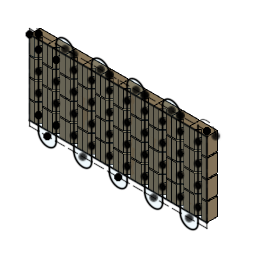
model (Autodesk Fusion 360 design; units mm, degrees)
Autodesk Fusion 360 part; units mm, degrees
sketch "profile" plane through (0, 0, 0) normal (0, 0, 1) x (1, 0, 0) in component "rail"
  line L0 (0, 0) -> (30, 0)
  line L1 (30, 0) -> (30, -18)
  line L2 (0, -18) -> (0, 0)
  line L3 (8.75, -18) -> (15, -11.75)
  line L4 (15, -11.75) -> (21.25, -18)
  line L5 (30, -18) -> (21.25, -18)
  line L6 (8.75, -18) -> (0, -18)
  line L7 (11.825, -14.925) -> (11.825, -8.575)
  line L8 (11.825, -8.575) -> (18.175, -8.575)
  line L9 (18.175, -8.575) -> (18.175, -14.925)
  line L10 (15, -11.75) -> (15, -8.575) construction
  line L11 (8.75, -18) -> (15, -18) construction
  line L12 (15, -18) -> (21.25, -18) construction
  circle A0 centre (15, -15.9926) radius 3 construction
  dimension "d4" = 30
  dimension "d6" = 3.175
  dimension "d8" = 18
  dimension "d9" = 6.35
  dimension "d25" = 12.5
  dimension "d26" = 6.25
  dimension "d27" = 6
  dimension "d28" = 15.9926
  dimension "d29" = 9.425
  constraint horizontal L0
  constraint vertical L1
  constraint horizontal L5
  constraint vertical L2
  constraint coincident L0.start L2.end
  constraint coincident L3.start L5
  constraint perpendicular L3 L4
  constraint collinear L5 L6
  constraint equal L5 L6
  constraint equal L3 L4
  constraint coincident L3 L7.start
  constraint coincident L4 L9.end
  constraint vertical L7
  constraint vertical L9
  constraint horizontal L8
  constraint midpoint L8 L10.end
  constraint vertical L10
  constraint horizontal L11
  constraint horizontal L12
  constraint equal L11 L12
  constraint tangent L3 A0
  constraint tangent L4 A0
  measures "d4" distance of L0.start L0.end
  measures "d6" vertical distance of L3.end L10.end
  measures "d8" distance of L0.start L2.start
  measures "d9" distance of L7 L9
  measures "d25" distance of L3.start L4.end
  measures "d26" distance of L3.end L11.end
  measures "d27" diameter of A0
  measures "d28" distance of L0 A0.centre
  measures "d29" distance of L6 L8
extrude "Extrude1" add sketch "profile" along normal blind 30 makes body 1 in component "rail"
sketch "hole" plane through (0, 0, 0) normal (0, 1, 0) x (-1, 0, 0) in component "rail"
  line L0 (-30, 0) -> (0, 0)
  line L1 (0, 0) -> (0, 30)
  line L2 (0, 30) -> (-30, 30)
  line L3 (-30, 30) -> (-30, 0)
  line L4 (-30, 0) -> (0, 30) construction
  circle A0 centre (-15, 15) radius 3.175
  dimension "d13" = 6.35
  constraint coincident L0.start L3.end
  constraint coincident L1.end L2.start
  constraint midpoint L4 A0.centre
  measures "d13" diameter of A0
ref_plane "WorkPlane1" through (15, -11.75, 15) normal (0, 1, 0) x (0, 0, 1) in component "rail"
extrude "Extrude2" cut sketch "hole" along normal blind 3.175 and the other way blind 30 from surface at -11.75 contours A0 bodies 1 in component "rail"
pattern_linear "R-Pattern1" count 10 spacing 30 along (1, 0, 0) count 4 spacing 32 along (0, 0, -1) of bodies 1 makes body 2 at (40, 0, 10) makes body 3 at (70, 0, 10) makes body 4 at (100, 0, 10) makes body 5 at (130, 0, 10) makes body 6 at (160, 0, 10) makes body 7 at (190, 0, 10) makes body 8 at (220, 0, 10) makes body 9 at (250, 0, 10) makes body 10 at (280, 0, 10) makes body 11 at (10, 0, -22) makes body 12 at (40, 0, -22) makes body 13 at (70, 0, -22) makes body 14 at (100, 0, -22) makes body 15 at (130, 0, -22) makes body 16 at (160, 0, -22) makes body 17 at (190, 0, -22) makes body 18 at (220, 0, -22) makes body 19 at (250, 0, -22) makes body 20 at (280, 0, -22) makes body 21 at (10, 0, -54) makes body 22 at (40, 0, -54) makes body 23 at (70, 0, -54) makes body 24 at (100, 0, -54) makes body 25 at (130, 0, -54) makes body 26 at (160, 0, -54) makes body 27 at (190, 0, -54) makes body 28 at (220, 0, -54) makes body 29 at (250, 0, -54) makes body 30 at (280, 0, -54) makes body 31 at (10, 0, -86) makes body 32 at (40, 0, -86) makes body 33 at (70, 0, -86) makes body 34 at (100, 0, -86) makes body 35 at (130, 0, -86) makes body 36 at (160, 0, -86) makes body 37 at (190, 0, -86) makes body 38 at (220, 0, -86) makes body 39 at (250, 0, -86) makes body 40 at (280, 0, -86) in component "rail"
sketch "Sketch1" plane through (0, -18, 0) normal (0, -1, 0) x (1, 0, 0)
  line L0 (0, 0) -> (8.75, 0)
  line L1 (8.75, 0) -> (8.75, 30)
  line L2 (8.75, 30) -> (0, 30)
  line L3 (0, 30) -> (0, 0)
  arc A0 (15, 18.175) -> (15, 11.825) centre (15, 15) ccw
  arc A1 (15, 11.825) -> (15, 18.175) centre (15, 15) ccw
  circle A2 centre (15, 15) radius 3.1782
  circle A3 centre (45, 15) radius 3.1782
  circle A4 centre (75, 15) radius 3.1782
  circle A5 centre (105, 15) radius 3.1782
  circle A6 centre (135, 15) radius 3.1782
  circle A7 centre (165, 15) radius 3.1782
  circle A8 centre (195, 15) radius 3.1782
  circle A9 centre (225, 15) radius 3.1782
  circle A10 centre (255, 15) radius 3.1782
  circle A11 centre (285, 15) radius 3.1782
  circle A12 centre (15, -17) radius 3.1782
  circle A13 centre (45, -17) radius 3.1782
  circle A14 centre (75, -17) radius 3.1782
  circle A15 centre (105, -17) radius 3.1782
  circle A16 centre (135, -17) radius 3.1782
  circle A17 centre (165, -17) radius 3.1782
  circle A18 centre (195, -17) radius 3.1782
  circle A19 centre (225, -17) radius 3.1782
  circle A20 centre (255, -17) radius 3.1782
  circle A21 centre (285, -17) radius 3.1782
  circle A22 centre (15, -49) radius 3.1782
  circle A23 centre (45, -49) radius 3.1782
  circle A24 centre (75, -49) radius 3.1782
  circle A25 centre (105, -49) radius 3.1782
  circle A26 centre (135, -49) radius 3.1782
  circle A27 centre (165, -49) radius 3.1782
  circle A28 centre (195, -49) radius 3.1782
  circle A29 centre (225, -49) radius 3.1782
  circle A30 centre (255, -49) radius 3.1782
  circle A31 centre (285, -49) radius 3.1782
  circle A32 centre (15, -81) radius 3.1782
  circle A33 centre (45, -81) radius 3.1782
  circle A34 centre (75, -81) radius 3.1782
  circle A35 centre (105, -81) radius 3.1782
  circle A36 centre (135, -81) radius 3.1782
  circle A37 centre (165, -81) radius 3.1782
  circle A38 centre (195, -81) radius 3.1782
  circle A39 centre (225, -81) radius 3.1782
  circle A40 centre (255, -81) radius 3.1782
  circle A41 centre (285, -81) radius 3.1782
  line L4 (15, 38.35) -> (15, -104.35)
  line L5 (45, 38.35) -> (45, -104.35)
  arc A42 (15, -104.35) -> (45, -104.35) centre (30, -104.35) ccw
  circle A43 centre (15, 38.35) radius 6.35 construction
  line L6 (45, 38.35) -> (75, 38.35) construction
  arc A44 (75, 38.35) -> (45, 38.35) centre (60, 38.35) ccw
  line L7 (75, 38.35) -> (75, -104.35)
  arc A45 (75, -104.35) -> (105, -104.35) centre (90, -104.35) ccw
  line L8 (105, 38.35) -> (105, -104.35)
  arc A46 (135, 38.35) -> (105, 38.35) centre (120, 38.35) ccw
  line L9 (135, 38.35) -> (135, -104.35)
  arc A47 (135, -104.35) -> (165, -104.35) centre (150, -104.35) ccw
  line L10 (165, 38.35) -> (165, -104.35)
  arc A48 (195, 38.35) -> (165, 38.35) centre (180, 38.35) ccw
  line L11 (195, 38.35) -> (195, -104.35)
  arc A49 (195, -104.35) -> (225, -104.35) centre (210, -104.35) ccw
  line L12 (225, 38.35) -> (225, -104.35)
  arc A50 (255, 38.35) -> (225, 38.35) centre (240, 38.35) ccw
  line L13 (255, 38.35) -> (255, -104.35)
  arc A51 (255, -104.35) -> (285, -104.35) centre (270, -104.35) ccw
  line L14 (285, 38.35) -> (285, -104.35)
  arc A52 (315, 38.35) -> (285, 38.35) centre (300, 38.35) ccw construction
  line L15 (0, -104.35) -> (300, -104.35) construction
  line L16 (300, -104.35) -> (300, 38.35) construction
  line L17 (300, 38.35) -> (0, 38.35) construction
  line L18 (0, 38.35) -> (0, -104.35) construction
  line L19 (0, 30) -> (300, 30)
  line L20 (0, -96) -> (300, -96)
  line L21 (150, 30) -> (150, 38.35) construction
  line L22 (150, -104.35) -> (150, -96) construction
  line L23 (0, 30) -> (0, -96)
  line L24 (300, -96) -> (300, 30)
  dimension "d32" = 30
  dimension "d33" = -32
  dimension "d34" = 6.3563
  dimension "d35" = 23.35
  dimension "d36" = 23.35
  dimension "d37" = 12.7
  dimension "d40" = 60
  dimension "d41" = 0
  constraint concentric A0 A2
  constraint coincident A0.centre L4
  constraint coincident A32.centre L4
  constraint coincident A3.centre L5
  constraint coincident A33.centre L5
  constraint tangent L4 A42
  constraint tangent L5 A42
  constraint equal L4 L5
  constraint coincident L4.start A43.centre
  constraint perpendicular L5 L6
  constraint tangent L5 A44
  constraint equal A42 A44
  constraint horizontal L15
  constraint vertical L16
  constraint horizontal L17
  constraint vertical L18
  constraint coincident A52.centre L16.end
  constraint coincident A42.centre L15
  constraint coincident L0.start L18
  constraint coincident L2.end L3.start
  constraint coincident L16 L19.end
  constraint coincident L18 L20.start
  constraint coincident L16 L20.end
  constraint horizontal L19
  constraint horizontal L20
  constraint midpoint L19 L21.start
  constraint midpoint L17 L21.end
  constraint coincident A47.centre L22.start
  constraint midpoint L20 L22.end
  constraint equal L21 L22
  measures "d34" diameter of A2
  measures "d35" distance of A32.centre L4.end
  measures "d36" distance of A0.centre L4.start
  measures "d37" diameter of A43
component "rail" placed x (1, 0, 0) y (0, 1, 0) z (0, 0, 1) at (0, 0, 0)
equation "spacing = 30 mm"
equation "height = 30 mm"
equation "magDiameter = 1/4\""
equation "d4 = spacing"
equation "magDepth = 1/8\""
equation "d6 = magDepth"
equation "d9 = magDiameter"
equation "d11 = height"
equation "d13 = magDiameter"
equation "d16 = magDepth"
equation "d22 = spacing"
equation "d23 = -( spacing + 2 mm )"
equation "d32 = spacing"
equation "d33 = -( spacing + 2 mm )"
equation "d34 = 1/4\" * 1.001"
equation "d35 = spacing / 2 + 1/4\" + 2 mm"
equation "d36 = d35"
equation "d37 = 1/2\""
equation "d40 = 2 * spacing"
